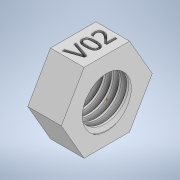
# Autodesk Inventor part: 1bThreads5_8x11InternalNut-V02
Saved by Autodesk Inventor 2021.1 (Build 251245010, 245A)
## iProperties
Created: 2020-10-17
Part Number: 1bThreads5_8x11InternalNut-V02
Material: Generic
Document SubType Name: Modeling
Designer: robst
Density: 1 g/cm^3
Appearance: Default
Author: robst
Autodesk Inventor part; units mm, degrees
ref_plane "YZ Plane" through (0, 0, 0) normal (1, 0, 0) x (0, 1, 0)
ref_plane "XZ Plane" through (0, 0, 0) normal (0, 1, 0) x (-1, 0, 0)
ref_plane "XY Plane" through (0, 0, 0) normal (0, 0, 1) x (1, 0, 0)
sketch "1bInternalThreadSketch" plane through (0, 0, 0) normal (0, 0, 1) x (1, 0, 0)
  line L0 (-1.0578, 8.2398) -> (20.6866, 8.2398) construction
  line L1 (10.6977, 6.9342) -> (11.3057, 6.9342) construction
  line L2 (-1.0578, 8.2398) -> (-0.304, 6.9342)
  line L3 (-0.304, 6.9342) -> (0.304, 6.9342)
  line L4 (0.304, 6.9342) -> (1.0094, 8.1559)
  line L5 (1.2997, 8.1559) -> (2.0051, 6.9342)
  arc A0 (1.2997, 8.1559) -> (1.0094, 8.1559) centre (1.1545, 8.0721) ccw
  line L6 (-1.0578, 8.2398) -> (-1.0578, 6.9621) construction
  line L7 (2.0051, 6.9342) -> (2.6131, 6.9342)
  line L8 (2.6131, 6.9342) -> (3.3185, 8.1559)
  line L9 (3.6088, 8.1559) -> (4.3187, 6.9264)
  arc A1 (3.6088, 8.1559) -> (3.3185, 8.1559) centre (3.4636, 8.0721) ccw
  line L10 (4.3187, 6.9264) -> (4.3142, 6.9342)
  line L11 (4.3142, 6.9342) -> (4.9222, 6.9342)
  line L12 (4.9222, 6.9342) -> (5.6275, 8.1559)
  line L13 (5.9179, 8.1559) -> (6.1974, 7.6718)
  arc A2 (5.9179, 8.1559) -> (5.6275, 8.1559) centre (5.7727, 8.0721) ccw
  line L14 (6.1974, 7.6718) -> (6.6233, 6.9342)
  line L15 (0, 0) -> (0, 8.2398) construction
  line L16 (0.304, 6.9342) -> (2.0051, 6.9342)
  point P0 (1.1545, 8.2398)
  point P1 (3.4636, 8.2398)
  dimension "d141" = 6.9342
  dimension "d142" = 8.2398
  dimension "d148" = 0.1676
  dimension "d150" = 60
  dimension "d151" = 30
  dimension "d154" = 0.1676
  dimension "d155" = 60
  dimension "d158" = 2.3091
  dimension "d168" = 60
  dimension "d169" = 0.1676
  dimension "d173" = 2.3091
  dimension "d175" = 60
  dimension "d176" = 60
  dimension "d177" = 60
  dimension "d178" = 0.608
  dimension "d179" = 0.608
  dimension "d180" = 0.608
  dimension "d181" = 1.1545
  constraints: 32 end point, 9 tangent, 8 point on circle, 4 collinear, 3 centre point, 3 horizontal, 1 perpendicular, 1 point on line, 1 vertical, 10 other
  measures "d142" distance from line of L0 L15.start
  measures "d148" radius of A0
  measures "d150" angle of L4 L2
  measures "d151" angle of L2 L6
  measures "d154" radius of A1
  measures "d155" angle of L8 L5
  measures "d158" distance of A1.centre A0.centre
  measures "d168" angle of L12 L9
  measures "d169" radius of A2
  measures "d173" distance of A2.centre A1.centre
  measures "d175" angle of L5 L4
  measures "d176" angle of L9 L8
  measures "d177" angle of L14 L12
  measures "d178" distance of L3.end L2.end
  measures "d179" distance of L7.end L5.end
  measures "d180" distance of L11.end L10.end
  measures "d181" distance from line of A0.centre L15
sketch "Sketch9" plane through (0, 0, 0) normal (0, 0, 1) x (1, 0, 0)
  line L0 (1.1545, 8.0886) -> (3.4636, 8.0886) projected
  line L1 (-1.0578, 8.2398) -> (20.6866, 8.2398) construction
  line L2 (0, 0) -> (0, 8.2398) construction
  line L3 (-0.304, 6.9342) -> (0.304, 6.9342) projected
  line L4 (0, 6.9342) -> (-10.16, 6.9342)
  line L5 (-10.16, 6.9342) -> (-10.16, 10.7798)
  line L6 (-10.16, 10.7798) -> (0, 10.7798)
  line L7 (0, 10.7798) -> (0, 6.9342)
  line L8 (-16.3293, 0) -> (26.8559, 0) projected
  point P0 (1.1545, 8.2398)
  point P1 (3.4636, 8.2398)
  dimension "d182" = 10.16
  dimension "d183" = 10.7798
  constraints: 8 end point, 2 parallel, 1 horizontal, 1 midpoint, 1 perpendicular
  measures "d182" distance of L5.end L6.end
  measures "d183" distance from line of L6 point (0, 0)
revolve "Revolution2" add sketch "Sketch9" angle 360 about axis through (-10, 0, 0) along (1, 0, 0)
coil "Coil3" sketch "1bInternalThreadSketch" operation cut axis through (-10, 0, 0) along (-1, 0, 0) pitch 2.3091 turns 6.4 hand right
sketch "Sketch10" plane through (-10.16, 0, 0) normal (-1, 0, 0) x (0, 0, 1)
  line L0 (-6.8741, 11.9062) -> (6.8741, 11.9063)
  line L1 (6.8741, 11.9063) -> (13.7482, 0)
  line L2 (13.7482, 0) -> (6.8741, -11.9062)
  line L3 (6.8741, -11.9062) -> (-6.8741, -11.9062)
  line L4 (-6.8741, -11.9062) -> (-13.7482, 0)
  line L5 (-13.7482, 0) -> (-6.8741, 11.9062)
  circle A0 centre (0, 0) radius 10.635
  dimension "d193" = 23.8125
  constraints: 12 end point, 2 coincident, 1 centre point, 1 horizontal, 13 other
  measures "d193" distance between parallel lines of L3 L0
extrude "Extrusion5" add sketch "Sketch10" against normal blind 10.16
sketch "Sketch11" plane through (-10.16, 11.9063, 6.8741) normal (0, 1, 0) x (1, 0, 0)
  line L0 (0, 0) -> (10.16, 0) construction
  line L1 (5.08, 0) -> (5.08, 13.7482) construction
  line L2 (0, 13.7482) -> (10.16, 13.7482) construction
  line L3 (2.54, 5.1759) -> (7.62, 3.4263)
  line L4 (7.62, 3.4263) -> (7.62, 2.6977)
  line L5 (7.62, 2.6977) -> (2.54, 0.9481)
  line L6 (2.54, 0.9481) -> (2.54, 1.6726)
  line L7 (2.54, 1.6726) -> (6.7596, 3.0805)
  line L8 (6.7596, 3.0805) -> (2.54, 4.4885)
  line L9 (2.54, 4.4885) -> (2.54, 5.1759)
  spline S0 degree 2 poles (5.08, 8.7369) (6.4467, 8.7369) (7.727, 7.9424) (7.727, 7.1149) knots 0 0 0 1 2 2 2
  spline S1 degree 2 poles (7.727, 7.1149) (7.727, 6.2751) (6.422, 5.4888) (5.0841, 5.4888) knots 0 0 0 1 2 2 2
  spline S2 degree 2 poles (5.0841, 5.4888) (3.7091, 5.4888) (2.4371, 6.2833) (2.4371, 7.1149) knots 0 0 0 1 2 2 2
  spline S3 degree 2 poles (2.4371, 7.1149) (2.4371, 7.9506) (3.7544, 8.7369) (5.08, 8.7369) knots 0 0 0 1 2 2 2
  spline S4 degree 2 poles (6.6279, 7.8641) (6.3768, 7.9629) (5.6028, 8.0453) (5.08, 8.0453) knots 0 0 0 1 2 2 2
  spline S5 degree 2 poles (5.08, 8.0453) (4.5572, 8.0453) (3.7874, 7.9629) (3.528, 7.86) knots 0 0 0 1 2 2 2
  spline S6 degree 2 poles (3.528, 7.86) (3.2687, 7.7571) (3.0011, 7.399) (3.0011, 7.1149) knots 0 0 0 1 2 2 2
  spline S7 degree 2 poles (3.0011, 7.1149) (3.0011, 6.8309) (3.2687, 6.4645) (3.5362, 6.3574) knots 0 0 0 1 2 2 2
  spline S8 degree 2 poles (3.5362, 6.3574) (3.7956, 6.2545) (4.586, 6.1804) (5.0841, 6.1804) knots 0 0 0 1 2 2 2
  spline S9 degree 2 poles (5.0841, 6.1804) (5.6193, 6.1804) (6.3356, 6.2463) (6.6155, 6.3533) knots 0 0 0 1 2 2 2
  spline S10 degree 2 poles (6.6155, 6.3533) (6.879, 6.4521) (7.163, 6.8185) (7.163, 7.1149) knots 0 0 0 1 2 2 2
  spline S11 degree 2 poles (7.163, 7.1149) (7.163, 7.3948) (6.8955, 7.7612) (6.6279, 7.8641) knots 0 0 0 1 2 2 2
  line L10 (7.62, 12.5201) -> (7.62, 9.3873)
  line L11 (7.62, 9.3873) -> (6.8996, 9.3873)
  spline S12 degree 2 poles (6.8996, 9.3873) (6.5826, 9.7249) (5.9939, 10.3259) (5.6769, 10.6141) knots 0 0 0 1 2 2 2
  spline S13 degree 2 poles (5.6769, 10.6141) (5.0388, 11.1945) (4.2731, 11.6186) (3.8656, 11.6186) knots 0 0 0 1 2 2 2
  spline S14 degree 2 poles (3.8656, 11.6186) (3.6515, 11.6186) (3.3304, 11.4868) (3.2275, 11.3674) knots 0 0 0 1 2 2 2
  spline S15 degree 2 poles (3.2275, 11.3674) (3.1246, 11.2481) (3.0217, 10.9352) (3.0217, 10.7458) knots 0 0 0 1 2 2 2
  spline S16 degree 2 poles (3.0217, 10.7458) (3.0217, 10.5647) (3.1122, 10.1942) (3.1822, 10.0254) knots 0 0 0 1 2 2 2
  spline S17 degree 2 poles (3.1822, 10.0254) (3.2398, 9.8813) (3.4045, 9.6137) (3.4621, 9.5314) knots 0 0 0 1 2 2 2
  line L12 (3.4621, 9.5314) -> (3.4621, 9.4944)
  line L13 (3.4621, 9.4944) -> (2.7376, 9.4944)
  spline S18 degree 2 poles (2.7376, 9.4944) (2.6347, 9.7043) (2.433, 10.4577) (2.433, 10.7952) knots 0 0 0 1 2 2 2
  spline S19 degree 2 poles (2.433, 10.7952) (2.433, 11.5074) (3.1863, 12.3102) (3.8285, 12.3102) knots 0 0 0 1 2 2 2
  spline S20 degree 2 poles (3.8285, 12.3102) (4.129, 12.3102) (4.6313, 12.1702) (4.8453, 12.0467) knots 0 0 0 1 2 2 2
  spline S21 degree 2 poles (4.8453, 12.0467) (5.0676, 11.9232) (5.504, 11.565) (5.714, 11.3674) knots 0 0 0 1 2 2 2
  spline S22 degree 2 poles (5.714, 11.3674) (6.0639, 11.0463) (6.8131, 10.2601) (7.0313, 10.0254) knots 0 0 0 1 2 2 2
  line L14 (7.0313, 10.0254) -> (7.0313, 12.5201)
  line L15 (7.0313, 12.5201) -> (7.62, 12.5201)
  point P0 (10.16, 6.8741)
  constraints: 2 end point, 2 midpoint, 1 vertical
extrude "Extrusion6" cut sketch "Sketch11" against normal blind 1.27
equation "\"d141\" = b1MinorRadius"
equation "\"d142\" = b1MajorRadius"
equation "\"d148\" = b1RootRadius"
equation "\"d150\" = threadAngle"
equation "\"d151\" = 0.5 * threadAngle"
equation "\"d154\" = b1RootRadius"
equation "\"d155\" = threadAngle"
equation "\"d158\" = pitch"
equation "\"d168\" = threadAngle"
equation "\"d169\" = b1RootRadius"
equation "\"d175\" = threadAngle"
equation "\"d176\" = threadAngle"
equation "\"d177\" = threadAngle"
equation "\"d181\" = 0.5 * pitch"
equation "\"d185\" = pitch"
equation "\"d193\" = nutExternalHexSize"
equation "\"threadAngle\" = 60deg"
equation "\"b1MajorDiameter\" = 16.47952"
equation "\"b1MajorRadius\" = 0.5 * b1MajorDiameter"
equation "\"b1MinorDiameter\" = 13.8684"
equation "\"b1RootRadius\" = 0.16764"
equation "\"b1MinorRadius\" = 0.5 * b1MinorDiameter"
equation "\"b1ThreadDepth\" = 1.27762"
equation "\"b1CrestFlat\" = 0.64008"
equation "\"nutExternalHexSize\" = 23.8125"
equation "\"b1CrestRadiusMax\" = 0"
equation "\"pitch\" = 2.309091"
body "Solid3"
